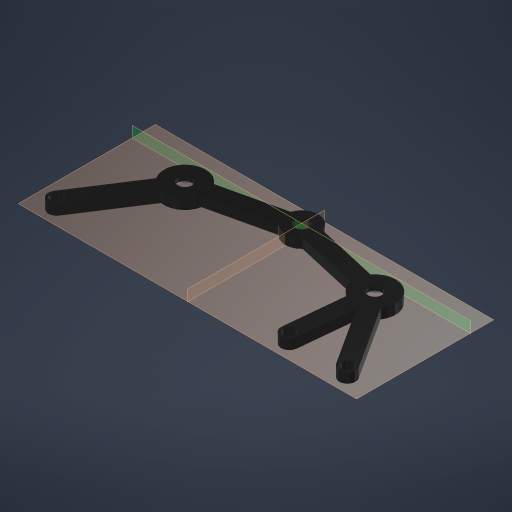
# Autodesk Inventor part: PD_Sensor
Saved by Autodesk Inventor 2024 (Build 280153000, 153)
## iProperties
Manager: Louis Van Roosmaelen
Company: DCS - DIGITAL COMBAT SIMULATOR
Created: 2023-12-25
Part Number: PD_Sensor
Material: S235
Catalog Web Link: http://emmausbovenbouw.op-weg.be/
Vendor: Emmaüsinstituut Bovenbouw Aalter
Document SubType Name: Modeling
Designer: Louis
Engineer: Declercq St.
Manufacturer: Standard
Standards Organization: Custom
Density: 7.86 g/cm^3
Appearance: Smooth - Black
IDENT.NR.: AJ2022
TEAM: 30
Title: F18C Home Cockpit
Author: Louis
Keywords: Ø
Autodesk Inventor part; units mm, degrees
sketch "Sketch1" plane through (0, 0, 0) normal (0, 0, 1) x (1, 0, 0)
  line L0 (0, 1.6506) -> (0, -1.6506) construction
  line L1 (-3.3363, 0) -> (3.3363, 0) construction
  circle A0 centre (-22.86, -5.25) radius 2
  circle A1 centre (22.86, -5.25) radius 2
  circle A2 centre (0, 0) radius 2
  circle A3 centre (-35, -24) radius 2
  circle A4 centre (21, -24) radius 2
  circle A5 centre (35, -24) radius 2
  line L2 (-36.6788, -22.913) -> (-24.5388, -4.163)
  line L3 (-21.1812, -6.337) -> (-33.3212, -25.087)
  line L4 (33.3212, -25.087) -> (21.1812, -6.337)
  line L5 (24.5388, -4.163) -> (36.6788, -22.913)
  line L6 (23.3077, -3.3007) -> (0.4477, 1.9493)
  line L7 (-22.4123, -7.1993) -> (0.4477, -1.9493)
  line L8 (-23.3077, -3.3007) -> (-0.4477, 1.9493)
  line L9 (-0.4477, -1.9493) -> (22.4123, -7.1993)
  line L10 (19.0098, -23.8026) -> (20.8698, -5.0526)
  line L11 (22.9902, -24.1974) -> (24.8502, -5.4474)
  point P0 (19.0231, -24.3028)
  point P1 (1.0254, -1.7172)
  point P2 (-21.6219, -7.0177)
  point P3 (0, 3.0781)
  point P4 (22.9979, -23.9085)
  point P5 (21.6219, -7.0177)
  point P6 (24.2863, -11.1327)
  point P7 (20.6959, -6.8051)
  dimension "d0" = 45.72
  dimension "d1" = 22.86
  dimension "d4" = 4
  dimension "d5" = 4
  dimension "d6" = 4
  dimension "d7" = 18.75
  dimension "d8" = 18.75
  dimension "d9" = 14
  dimension "d10" = 18.75
  dimension "d11" = 56
  dimension "d12" = 70
  dimension "d13" = 35
  dimension "d14" = 4
  dimension "d15" = 4
  dimension "d16" = 4
  dimension "d34" = 5.25
  dimension "d35" = 5.25
  constraints: 24 end point, 23 point on circle, 20 tangent, 8 coincident, 6 centre point, 2 midpoint, 1 horizontal, 1 vertical
  measures "d0" distance of point (-22.86, -5.25) point (22.86, -5.25)
  measures "d1" horizontal distance of point (-22.86, -5.25) point (0, 0)
  measures "d4" diameter of A0
  measures "d5" diameter of A1
  measures "d6" diameter of A2
  measures "d7" vertical distance of point (22.86, -5.25) point (35, -24)
  measures "d8" vertical distance of point (-35, -24) A0.centre
  measures "d9" distance of point (35, -24) point (21, -24)
  measures "d10" vertical distance of point (-22.86, -5.25) point (21, -24)
  measures "d11" distance of point (21, -24) point (-35, -24)
  measures "d12" distance of point (35, -24) point (-35, -24)
  measures "d13" horizontal distance of point (0, 0) point (35, -24)
  measures "d14" diameter of A3
  measures "d15" diameter of A4
  measures "d16" diameter of A5
  measures "d34" vertical distance of point (0, 0) point (-22.86, -5.25)
  measures "d35" vertical distance of point (0, 0) point (22.86, -5.25)
extrude "Extrusion1" add sketch "Sketch1" along normal blind 2.4
sketch "Sketch2" plane through (0, 0, 2.4) normal (0, 0, 1) x (1, 0, 0)
  line L0 (-21.6219, -7.0177) -> (-33.3212, -25.087) projected
  arc A0 (-36.6788, -22.913) -> (-33.3212, -25.087) centre (-35, -24) ccw projected
  line L1 (-36.6788, -22.913) -> (-24.5388, -4.163) projected
  arc A1 (-23.3077, -3.3007) -> (-24.5388, -4.163) centre (-22.86, -5.25) ccw projected
  line L2 (-23.3077, -3.3007) -> (-0.4477, 1.9493) projected
  line L3 (24.5388, -4.163) -> (36.6788, -22.913) projected
  arc A2 (33.3212, -25.087) -> (36.6788, -22.913) centre (35, -24) ccw projected
  line L4 (33.3212, -25.087) -> (24.2863, -11.1327) projected
  line L5 (0, -2.0521) -> (-21.6219, -7.0177) projected
  arc A3 (19.0098, -23.8026) -> (22.9902, -24.1974) centre (21, -24) ccw projected
  line L6 (0.4477, 1.9493) -> (23.3077, -3.3007) projected
  arc A4 (24.5388, -4.163) -> (23.3077, -3.3007) centre (22.86, -5.25) ccw projected
  arc A5 (0.4477, 1.9493) -> (-0.4477, 1.9493) centre (0, 0) ccw projected
  line L7 (20.6959, -6.8051) -> (0, -2.0521) projected
  line L8 (24.2863, -11.1327) -> (22.9902, -24.1974) projected
  line L9 (19.0098, -23.8026) -> (20.6959, -6.8051) projected
  constraints: 3 coincident
hole "Hole1" at (-35, -24, 2.4) at (21, -24, 2.4) at (35, -24, 2.4) direction (0, 0, -1) diameter 2.8 depth 2.4
sketch "Sketch3" plane through (0, 0, 2.4) normal (0, 0, 1) x (1, 0, 0)
  circle A0 centre (35, -24) radius 1.4 projected
  circle A1 centre (21, -24) radius 1.4 projected
  circle A2 centre (-35, -24) radius 1.4 projected
  line L0 (-21.6219, -7.0177) -> (-33.3212, -25.087) projected
  arc A3 (-36.6788, -22.913) -> (-33.3212, -25.087) centre (-35, -24) ccw projected
  line L1 (-36.6788, -22.913) -> (-24.5388, -4.163) projected
  arc A4 (-23.3077, -3.3007) -> (-24.5388, -4.163) centre (-22.86, -5.25) ccw projected
  line L2 (-23.3077, -3.3007) -> (-0.4477, 1.9493) projected
  line L3 (24.5388, -4.163) -> (36.6788, -22.913) projected
  arc A5 (33.3212, -25.087) -> (36.6788, -22.913) centre (35, -24) ccw projected
  line L4 (33.3212, -25.087) -> (24.2863, -11.1327) projected
  line L5 (0, -2.0521) -> (-21.6219, -7.0177) projected
  arc A6 (19.0098, -23.8026) -> (22.9902, -24.1974) centre (21, -24) ccw projected
  line L6 (0.4477, 1.9493) -> (23.3077, -3.3007) projected
  arc A7 (24.5388, -4.163) -> (23.3077, -3.3007) centre (22.86, -5.25) ccw projected
  arc A8 (0.4477, 1.9493) -> (-0.4477, 1.9493) centre (0, 0) ccw projected
  line L7 (20.6959, -6.8051) -> (0, -2.0521) projected
  line L8 (24.2863, -11.1327) -> (22.9902, -24.1974) projected
  line L9 (19.0098, -23.8026) -> (20.6959, -6.8051) projected
  circle A9 centre (-22.86, -5.25) radius 5
  circle A10 centre (0, 0) radius 4
  circle A11 centre (22.86, -5.25) radius 5
  dimension "d36" = 10
  dimension "d37" = 8
  dimension "d38" = 10
  constraints: 7 coincident, 3 centre point
  measures "d36" diameter of A9
  measures "d37" diameter of A10
  measures "d38" diameter of A11
extrude "Extrusion3" add sketch "Sketch3" against normal up to surface (2.4 mm away) contours L5 A9 L0 | L0 A9 L1 A4 L2 L5 | A9 L2 A4 L1 | A10 L2 A8 L6 L7 L5 | L5 L7 A10 | A10 L6 A8 L2 | A11 L6 A7 L3 L9 L7 | L7 L9 A11 | A11 L3 A7 L6
sketch "Sketch4" plane through (0, 0, 0) normal (0, 0, -1) x (-1, 0, 0)
  arc A0 (-2.9285, -2.7246) -> (2.9285, -2.7246) centre (0, 0) ccw projected
  line L0 (-2.9285, -2.7246) -> (-17.946, -6.1735) projected
  arc A1 (-20.4174, -9.6128) -> (-17.946, -6.1735) centre (-22.86, -5.25) ccw projected
  line L1 (-20.4174, -9.6128) -> (-19.0098, -23.8026) projected
  arc A2 (-22.9902, -24.1974) -> (-19.0098, -23.8026) centre (-21, -24) ccw projected
  line L2 (-22.9902, -24.1974) -> (-24.2863, -11.1327) projected
  line L3 (-24.2863, -11.1327) -> (-33.3212, -25.087) projected
  arc A3 (-36.6788, -22.913) -> (-33.3212, -25.087) centre (-35, -24) ccw projected
  line L4 (-36.6788, -22.913) -> (-27.0294, -8.0097) projected
  arc A4 (-18.8414, -2.275) -> (-27.0294, -8.0097) centre (-22.86, -5.25) ccw projected
  line L5 (-18.8414, -2.275) -> (-3.8239, 1.1739) projected
  arc A5 (3.8239, 1.1739) -> (-3.8239, 1.1739) centre (0, 0) ccw projected
  line L6 (3.8239, 1.1739) -> (18.8414, -2.275) projected
  arc A6 (27.0294, -8.0097) -> (18.8414, -2.275) centre (22.86, -5.25) ccw projected
  line L7 (27.0294, -8.0097) -> (36.6788, -22.913) projected
  arc A7 (33.3212, -25.087) -> (36.6788, -22.913) centre (35, -24) ccw projected
  line L8 (33.3212, -25.087) -> (23.6718, -10.1837) projected
  arc A8 (17.946, -6.1735) -> (23.6718, -10.1837) centre (22.86, -5.25) ccw projected
  line L9 (17.946, -6.1735) -> (2.9285, -2.7246) projected
  circle A9 centre (-21, -24) radius 1.4 projected
  circle A10 centre (-35, -24) radius 1.4 projected
  circle A11 centre (35, -24) radius 1.4 projected
hole "Hole3" at (-22.86, -5.25, 0) at (22.86, -5.25, 0) direction (0, 0, 1) diameter 3.3 depth 2.4 countersink diameter 6 countersink angle 90
sketch "Sketch5" plane through (0, 0, 2.4) normal (0, 0, 1) x (1, 0, 0)
  circle A0 centre (22.86, -5.25) radius 1.65 projected
  circle A1 centre (-22.86, -5.25) radius 1.65 projected
  arc A2 (-2.9285, -2.7246) -> (2.9285, -2.7246) centre (0, 0) ccw projected
  line L0 (-2.9285, -2.7246) -> (-17.946, -6.1735) projected
  arc A3 (-23.6718, -10.1837) -> (-17.946, -6.1735) centre (-22.86, -5.25) ccw projected
  line L1 (-23.6718, -10.1837) -> (-33.3212, -25.087) projected
  arc A4 (-36.6788, -22.913) -> (-33.3212, -25.087) centre (-35, -24) ccw projected
  line L2 (-36.6788, -22.913) -> (-27.0294, -8.0097) projected
  arc A5 (-18.8414, -2.275) -> (-27.0294, -8.0097) centre (-22.86, -5.25) ccw projected
  line L3 (-18.8414, -2.275) -> (-3.8239, 1.1739) projected
  arc A6 (3.8239, 1.1739) -> (-3.8239, 1.1739) centre (0, 0) ccw projected
  line L4 (3.8239, 1.1739) -> (18.8414, -2.275) projected
  arc A7 (27.0294, -8.0097) -> (18.8414, -2.275) centre (22.86, -5.25) ccw projected
  line L5 (27.0294, -8.0097) -> (36.6788, -22.913) projected
  arc A8 (33.3212, -25.087) -> (36.6788, -22.913) centre (35, -24) ccw projected
  line L6 (33.3212, -25.087) -> (24.2863, -11.1327) projected
  line L7 (24.2863, -11.1327) -> (22.9902, -24.1974) projected
  arc A9 (19.0098, -23.8026) -> (22.9902, -24.1974) centre (21, -24) ccw projected
  line L8 (19.0098, -23.8026) -> (20.4174, -9.6128) projected
  arc A10 (17.946, -6.1735) -> (20.4174, -9.6128) centre (22.86, -5.25) ccw projected
  line L9 (17.946, -6.1735) -> (2.9285, -2.7246) projected
  circle A11 centre (21, -24) radius 1.4 projected
  circle A12 centre (35, -24) radius 1.4 projected
  circle A13 centre (-35, -24) radius 1.4 projected
hole "Hole4" at (0, 0, 2.4) direction (0, 0, -1) diameter 3.3 depth 2.4
equation "\"d8\" = d7"
equation "\"d10\" = d8"
equation "\"d13\" = 0.5 * d12"
equation "\"d35\" = d34"
body "Solid1"
